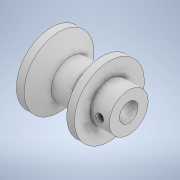
# Autodesk Inventor part: stepper_spool
Saved by Autodesk Inventor 2021 (Build 250183000, 183)
## iProperties
Created: 2021-06-16
Part Number: stepper_spool
Material: Generic
Document SubType Name: Modeling
Designer: Charlie
Density: 1 g/cm^3
Appearance: Default
Author: Charlie
Autodesk Inventor part; units mm, degrees
ref_plane "YZ Plane" through (0, 0, 0) normal (1, 0, 0) x (0, 1, 0)
ref_plane "XZ Plane" through (0, 0, 0) normal (0, 1, 0) x (-1, 0, 0)
ref_plane "XY Plane" through (0, 0, 0) normal (0, 0, 1) x (1, 0, 0)
sketch "Sketch1" plane through (0, 0, 0) normal (0, 0, 1) x (1, 0, 0)
  line L0 (0, 0) -> (20, 0)
  line L1 (0, 0) -> (0, 5)
  line L2 (0, 5) -> (0, 9)
  line L3 (0, 9) -> (2, 9)
  line L4 (20, 0) -> (20, 5)
  line L5 (20, 5) -> (0, 5)
  line L6 (15, 0) -> (15, 9)
  line L7 (15, 9) -> (13, 9)
  line L8 (13, 9) -> (10, 5)
  line L9 (2, 9) -> (13, 9) construction
  line L10 (7.5, 9) -> (7.5, -5.2368) construction
  line L11 (2, 9) -> (5, 5)
  point P0 (17.5, 0)
  point P1 (15, 5)
  dimension "d0" = 20
  dimension "d2" = 5
  dimension "d3" = 4
  dimension "d4" = 2
  dimension "d9" = 9
  dimension "d10" = 5
  dimension "d11" = 2
  dimension "d12" = 2.5
  dimension "d13" = 20
  constraints: 24 end point, 5 vertical, 2 horizontal, 2 midpoint, 2 point on line, 1 perpendicular, 1 symmetric about line
  measures "d0" distance of L0.start L0.end
  measures "d2" distance of L0.start L1.end
  measures "d3" distance of L1.end L2.end
  measures "d4" distance of L2.end L3.end
  measures "d9" distance of L6.start L6.end
  measures "d10" distance between parallel lines of L4 L6
  measures "d11" distance of L6.end L7.end
  measures "d12" distance from line of L4 point (17.5, 0)
  measures "d13" distance of L4.end L1.end
revolve "Revolution1" add sketch "Sketch1" angle 360 about axis through (0, 0, 0) along (1, 0, 0)
sketch "Sketch2" plane through (0, 0, 0) normal (-1, 0, 0) x (0, 0, 1)
  circle A0 centre (0, 0) radius 2.4
  dimension "d15" = 4.8
  constraints: 1 centre point, 1 coincident
  measures "d15" diameter of A0
extrude "Extrusion1" cut sketch "Sketch2" against normal blind 20
ref_plane "Work Plane1" through (20, 0, 0) normal (0, 0, -1) x (-1, 0, 0)
sketch "Sketch3" plane through (20, 0, 0) normal (0, 0, -1) x (-1, 0, 0)
  circle A0 centre (2.4908, 0) radius 1
  point P0 (20, 0)
  dimension "d18" = 2
  constraints: 1 centre point
  measures "d18" diameter of A0
extrude "Extrusion2" cut sketch "Sketch3" against normal blind 6
body "Solid1"
